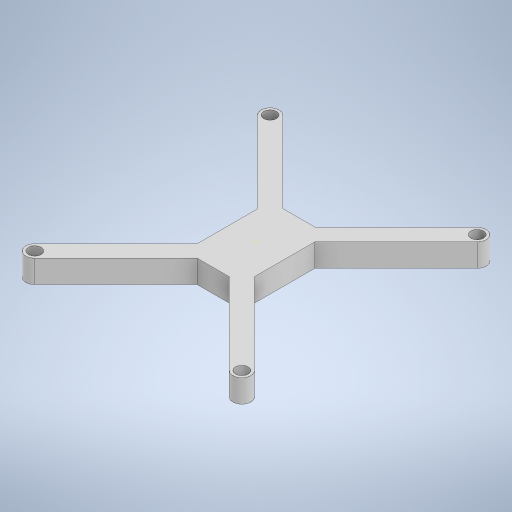
# Autodesk Inventor part: DrohneSkizze
Saved by Autodesk Inventor 2024.1 (Build 281209000, 209)
## iProperties
Created: 2023-11-26
Part Number: DrohneSkizze
Material: Generisch
Document SubType Name: Modeling
Designer: tobia
Density: 1 g/cm^3
Appearance: Vorgabe
Author: tobia
Autodesk Inventor part; units mm, degrees
ref_plane "YZ Plane" through (0, 0, 0) normal (1, 0, 0) x (0, 1, 0)
ref_plane "XZ Plane" through (0, 0, 0) normal (0, 1, 0) x (-1, 0, 0)
ref_plane "XY Plane" through (0, 0, 0) normal (0, 0, 1) x (1, 0, 0)
sketch "Skizze2" plane through (0, 0, 0) normal (0, 0, 1) x (1, 0, 0)
  line L0 (-50, 75) -> (50, 75)
  line L1 (50, 75) -> (50, -75)
  line L2 (50, -75) -> (-50, -75)
  line L3 (-50, -75) -> (-50, 75)
  line L4 (-28.5786, 75) -> (-170, 216.4214)
  line L5 (-170, 216.4214) -> (-192, 194.4214)
  line L6 (-192, 194.4214) -> (-50, 52.4214)
  circle A0 centre (-181, 205.4214) radius 15.5563
  line L7 (28.5786, 75) -> (170, 216.4214)
  line L8 (170, 216.4214) -> (192, 194.4214)
  line L9 (192, 194.4214) -> (50, 52.4214)
  line L10 (50, -53) -> (192, -195)
  line L11 (192, -195) -> (170, -217)
  line L12 (170, -217) -> (28, -75)
  line L13 (-50, -53) -> (-192, -195)
  line L14 (-192, -195) -> (-170, -217)
  line L15 (-170, -217) -> (-28, -75)
  circle A1 centre (181, -206) radius 15.5563
  circle A2 centre (181, 205.4214) radius 15.5563
  circle A3 centre (-181, -206) radius 15.5563
  point P0 (0, 0)
  point P1 (50, 0)
  point P2 (0, 75)
  dimension "d0" = 150
  dimension "d1" = 100
  dimension "d2" = 135
  dimension "d4" = 22
  dimension "d6" = 200
  dimension "d7" = 120
  dimension "d8" = 31.1127
  dimension "d9" = 135
  dimension "d10" = 0
  dimension "d12" = 22
  dimension "d14" = 200
  dimension "d15" = 120
  dimension "d16" = 135
  dimension "d17" = 22
  dimension "d20" = 120
  dimension "d21" = 120
  dimension "d22" = 22
  dimension "d23" = 120
  dimension "d24" = 135
  dimension "d25" = 120
  constraints: 32 end point, 8 perpendicular, 8 point on line, 6 midpoint, 3 centre point, 2 parallel, 1 horizontal, 1 horizontal alignment, 1 tangent, 1 vertical alignment, 3 other
  measures "d0" distance of L0.end L1.end
  measures "d1" distance of L0.start L0.end
  measures "d2" angle of L0 L4
  measures "d4" horizontal distance of L5.end L4.end
  measures "d6" distance from line of L4.start L5
  measures "d7" horizontal distance of L4.end L0.start
  measures "d8" diameter of A0
  measures "d9" angle of L7 L0
  measures "d10" angle of L7 L9
  measures "d12" horizontal distance of L7.end L8.end
  measures "d14" distance of L7.start L7.end
  measures "d15" distance from line of L1 L7.end
  measures "d16" angle of L1 L10
  measures "d17" horizontal distance of L10.end L11.end
  measures "d20" distance from line of L1 L11.end
  measures "d21" distance from line of L2 L10.end
  measures "d22" horizontal distance of L13.end L14.end
  measures "d23" distance from line of L3 L14.end
  measures "d24" angle of L2 L15
  measures "d25" distance from line of L2 L13.end
extrude "Extrusion1" add sketch "Skizze2" along normal blind 40
sketch "Skizze3" plane through (0, 0, 40) normal (0, 0, 1) x (1, 0, 0)
  arc A0 (-170, 216.4214) -> (-192, 194.4214) centre (-181, 205.4214) ccw projected
  circle A1 centre (-181, 205.4214) radius 11
  arc A2 (192, 194.4214) -> (170, 216.4214) centre (181, 205.4214) ccw projected
  circle A3 centre (181, 205.4214) radius 11
  arc A4 (170, -217) -> (192, -195) centre (181, -206) ccw projected
  circle A5 centre (181, -206) radius 11
  arc A6 (-192, -195) -> (-170, -217) centre (-181, -206) ccw projected
  circle A7 centre (-181, -206) radius 11
  point P0 (0, 0)
  dimension "d28" = 22
  dimension "d29" = 22
  dimension "d30" = 22
  dimension "d31" = 22
  constraints: 4 centre point, 4 coincident
  measures "d28" diameter of A1
  measures "d29" diameter of A3
  measures "d30" diameter of A5
  measures "d31" diameter of A7
extrude "Extrusion2" cut sketch "Skizze3" against normal blind 20
sketch "Skizze4" plane through (0, 0, 40) normal (0, 0, 1) x (1, 0, 0)
  point P0 (0, 0)
